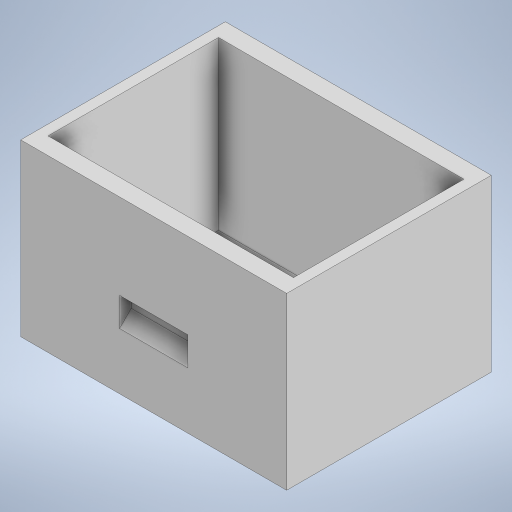
# Autodesk Inventor part: 容器
Saved by Autodesk Inventor 2023.1 (Build 271208000, 208)
## iProperties
Created: 2023-07-19
Part Number: 容器
Material: 常规
Document SubType Name: Modeling
Designer: Selcon
Density: 1 g/cm^3
Appearance: 默认
Author: Selcon
Autodesk Inventor part; units mm, degrees
ref_plane "YZ Plane" through (0, 0, 0) normal (1, 0, 0) x (0, 1, 0)
ref_plane "XZ Plane" through (0, 0, 0) normal (0, 1, 0) x (-1, 0, 0)
ref_plane "XY Plane" through (0, 0, 0) normal (0, 0, 1) x (1, 0, 0)
sketch "草图1" plane through (0, 0, 0) normal (0, 0, 1) x (1, 0, 0)
  line L0 (-195, 125) -> (195, 125)
  line L1 (195, 125) -> (195, -125)
  line L2 (195, -125) -> (-195, -125)
  line L3 (-195, -125) -> (-195, 125)
  line L4 (0, -175) -> (0, 175) projected
  line L5 (-273, 0) -> (273, 0) projected
  point P0 (0, 0)
  dimension "d0" = 250
  dimension "d1" = 390
  constraints: 8 end point, 2 parallel, 1 horizontal, 1 perpendicular, 2 other
  measures "d0" distance of L0.end L1.end
  measures "d1" distance of L0.start L0.end
extrude "拉伸1" add sketch "草图1" along normal mid plane 300
sketch "草图2" plane through (-195, 125, 150) normal (0, 1, 0) x (1, 0, 0)
  line L0 (15, 25) -> (375, 25)
  line L1 (375, 25) -> (375, 275)
  line L2 (375, 275) -> (15, 275)
  line L3 (15, 275) -> (15, 25)
  line L4 (-78, 150) -> (468, 150) projected
  line L5 (195, 360) -> (195, -60) projected
  point P0 (195, 150)
  dimension "d4" = 360
  dimension "d5" = 250
  constraints: 8 end point, 2 parallel, 1 horizontal, 1 perpendicular, 2 other
  measures "d4" distance of L1.end L2.end
  measures "d5" distance of L0.end L1.end
extrude "拉伸2" cut sketch "草图2" against normal blind 245
sketch "草图3" plane through (0, 0, 150) normal (0, 0, 1) x (1, 0, 0)
  line L0 (-50, 25) -> (50, 25)
  line L1 (50, 25) -> (50, -25)
  line L2 (50, -25) -> (-50, -25)
  line L3 (-50, -25) -> (-50, 25)
  line L4 (-273, 0) -> (273, 0) projected
  line L5 (0, -175) -> (0, 175) projected
  point P0 (0, 0)
  dimension "d8" = 100
  dimension "d9" = 50
  constraints: 8 end point, 2 parallel, 1 horizontal, 1 perpendicular, 2 other
  measures "d8" distance of L0.start L0.end
  measures "d9" distance of L0.end L1.end
extrude "拉伸3" cut sketch "草图3" against normal blind 17
sketch "草图4" plane through (0, 0, 150) normal (0, 0, 1) x (1, 0, 0)
  line L0 (-50, -25) -> (-50, 25) projected
  line L1 (50, 25) -> (50, -25) projected
  line L2 (-50, 25) -> (50, 25)
  line L3 (50, 25) -> (50, 0)
  line L4 (50, 0) -> (-50, 0)
  line L5 (-50, 0) -> (-50, 25)
  point P0 (0, 0)
  constraints: 8 end point, 2 parallel, 1 horizontal, 1 midpoint, 1 perpendicular
extrude "拉伸4" add sketch "草图4" against normal blind 5
mirror "镜像1" about plane through (0, 0, 0) normal (0, 0, 1) of "拉伸3", "拉伸4"
chamfer "倒角1" distance 17 angle 45 2 edges at (0, -25, 150) (0, -25, -150)
chamfer "倒角2" distance 5 angle 45 2 edges at (0, 0, 145) (0, 0, -145)
